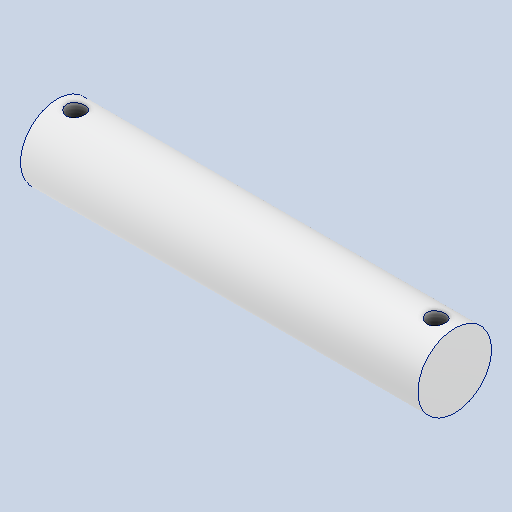
# Autodesk Inventor part: belt_liner_v1_shaft-54
Saved by Autodesk Inventor 2025.1 (Build 291241000, 241)
## iProperties
Created: 2024-12-08
Part Number: belt_liner_v1_shaft-54
Material: アルミニウム 6061
Document SubType Name: Modeling
Designer: haruy
Density: 2.7 g/cm^3
Appearance: アルミニウム - フラット
Author: haruy
Autodesk Inventor part; units mm, degrees
ref_plane "YZ Plane" through (0, 0, 0) normal (1, 0, 0) x (0, 1, 0)
ref_plane "XY Plane" through (0, 0, 0) normal (0, 0, 1) x (1, 0, 0)
sketch "スケッチ1" plane through (0, 0, 0) normal (1, 0, 0) x (0, 1, 0)
  circle A0 centre (0, 0) radius 5
  dimension "d0" = 10
  constraints: 1 centre point, 1 coincident
  measures "d0" diameter of A0
extrude "押し出し1" add sketch "スケッチ1" along normal blind 54
ref_plane "作業平面1" through (0, -5, 0) normal (0, 1, 0) x (-1, 0, 0)
sketch "スケッチ2" plane through (0, -5, 0) normal (0, 1, 0) x (-1, 0, 0)
  line L0 (0, 5) -> (0, -5) projected
  line L1 (-54, 5) -> (-54, -5) projected
  point P0 (0, 0)
  point P1 (-2.5, 0)
  point P2 (-51.5, 0)
  dimension "d3" = 2.5
  dimension "d4" = 2.5
  measures "d3" distance from line of L0 point (-2.5, 0)
  measures "d4" distance from line of L1 point (-51.5, 0)
hole "穴1" at (2.5, -5, 0) at (51.5, -5, 0) direction (0, 1, 0) diameter 2.5 end through all
thread "ねじ1" size "M2.5x0.45" class "6H" standard "ANSI Metric M Profile" full length
thread "ねじ2" size "M2.5x0.45" class "6H" standard "ANSI Metric M Profile" full length
